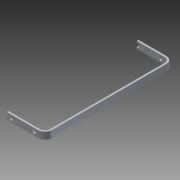
# Autodesk Inventor part: tie-together tier 1
Saved by Autodesk Inventor 2013 (Build 170138000, 138)
## iProperties
Created: 2013-01-24
Part Number: tie-together tier 1
Material: Aluminum 6061
Document SubType Name: Sheet Metal
Designer: Arpan
Density: 1 g/cm^3
Sheet Metal Rule: Default
Author: Arpan
Autodesk Inventor part; units mm, degrees
ref_plane "YZ Plane" through (0, 0, 0) normal (1, 0, 0) x (0, 1, 0)
ref_plane "XZ Plane" through (0, 0, 0) normal (0, 1, 0) x (-1, 0, 0)
ref_plane "XY Plane" through (0, 0, 0) normal (0, 0, 1) x (1, 0, 0)
sketch "Sketch1" plane through (0, 0, 0) normal (0, 0, 1) x (1, 0, 0)
  line L0 (0, 0) -> (-56.9976, 0)
  line L1 (-56.9976, 0) -> (-56.9976, 12.7)
  line L2 (-56.9976, 12.7) -> (0, 12.7)
  line L3 (0, 12.7) -> (0, 0)
  line L4 (0, 12.7) -> (-7.493, 12.7)
  line L5 (-7.493, 12.7) -> (-7.493, 6.35)
  line L6 (-56.9976, 12.7) -> (-49.5046, 12.7)
  line L7 (-49.5046, 12.7) -> (-49.5046, 6.35)
  circle A0 centre (-49.5046, 6.35) radius 3.302
  circle A1 centre (-7.493, 6.35) radius 3.302
  dimension "d1" = 56.9976
  dimension "d2" = 12.7
  dimension "d3" = 7.493
  dimension "d4" = 6.35
  dimension "d5" = 7.493
  dimension "d6" = 6.604
  dimension "d7" = 6.604
  dimension "d19" = 6.35
  measures "d1" distance of L0.start L0.end
  measures "d2" distance of L0.end L1.end
  measures "d3" distance of L2.end L4.end
  measures "d4" distance of L4.end L5.end
  measures "d5" distance of L1.end L6.end
  measures "d6" diameter of A0
  measures "d7" diameter of A1
  measures "d19" distance of L6.end L7.end
extrude "Plate1" add sketch "Sketch1" along normal blind 3.175
sketch "Sketch3" plane through (9.525, 0, -9.525) normal (1, 0, 0) x (0, 1, 0)
  line L0 (12.7, 0) -> (0, 0)
  line L1 (0, 0) -> (0, -208.2038)
  line L2 (0, -208.2038) -> (12.7, -208.2038)
  line L3 (12.7, -208.2038) -> (12.7, 0)
  constraints: 6 end point, 1 horizontal, 1 perpendicular, 1 vertical
edge flange "Flange2" height 220.9038 angle 90 thickness 3.175 bend radius 9.525 thickness toward (1, 0, 0) relief tear relief width 3.175 relief depth 1.5875 edges at (0, 6.35, 0) wall of the first edge with corners at (9.525, 12.7, -9.525) (9.525, 0, -9.525) (9.525, 0, -217.7288) (9.525, 12.7, -217.7288)
bend "Bend2"
corner "Corner2"
sketch "Sketch4" plane through (0, 0, -227.2538) normal (0, 0, -1) x (-1, 0, 0)
  line L0 (0, 12.7) -> (0, 0)
  line L1 (0, 0) -> (50.6476, 0)
  line L2 (50.6476, 0) -> (50.6476, 12.7)
  line L3 (50.6476, 12.7) -> (0, 12.7)
  constraints: 6 end point, 1 horizontal, 1 perpendicular, 1 vertical
edge flange "Flange3" height 63.3476 angle 90 thickness 3.175 bend radius 9.525 thickness toward (0, 0, -1) relief tear relief width 3.175 relief depth 1.5875 edges at (9.525, 6.35, -217.7288) wall of the first edge with corners at (0, 12.7, -227.2538) (0, 0, -227.2538) (-50.6476, 0, -227.2538) (-50.6476, 12.7, -227.2538)
bend "Bend3"
corner "Corner3"
sketch "Sketch5" plane through (0, 0, 3.175) normal (0, 0, 1) x (1, 0, 0)
  circle A0 centre (-7.493, 6.35) radius 3.302 projected
  circle A1 centre (-49.5046, 6.35) radius 3.302 projected
extrude "Extrusion1" cut sketch "Sketch5" against normal blind 2286
equation "\"d20\" = BendReliefWidth"
equation "\"d21\" = BendReliefDepth"
equation "\"d22\" = MinimumRemnant"
equation "\"d23\" = BendRadius"
equation "\"d27\" = CornerReliefSize"
equation "\"d28\" = GapSize"
equation "\"d29\" = JacobiRadiusSize"
equation "\"d30\" = BendReliefWidth"
equation "\"d31\" = BendReliefDepth"
equation "\"d32\" = MinimumRemnant"
equation "\"d33\" = BendRadius"
equation "\"d37\" = CornerReliefSize"
equation "\"d38\" = GapSize"
equation "\"d39\" = JacobiRadiusSize"
equation "\"BendRadius\" = Thickness"
equation "\"BendReliefWidth\" = Thickness"
equation "\"BendReliefDepth\" = 0.5 * Thickness"
equation "\"CornerReliefSize\" = 4 * Thickness"
equation "\"MinimumRemnant\" = 2 * Thickness"
equation "\"TransitionRadius\" = BendRadius"
equation "\"JacobiRadiusSize\" = BendRadius"
equation "\"GapSize\" = Thickness"
equation "\"d8\" = BendRadius"
equation "\"Thickness\" = 3.175"
body "Solid1"
